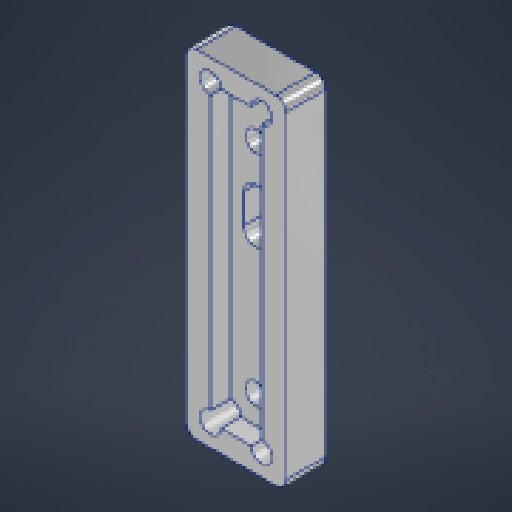
# Autodesk Inventor part: Zig
Saved by Autodesk Inventor 2024.3 (Build 283343000, 343)
## iProperties
Created: 2025-01-11
Part Number: Zig
Material: 알루미늄 6061
Document SubType Name: Modeling
Designer: ASUS
Density: 2.7 g/cm^3
Appearance: 알루미늄 - 평지
Author: ASUS
Autodesk Inventor part; units mm, degrees
ref_plane "YZ Plane" through (0, 0, 0) normal (1, 0, 0) x (0, 1, 0)
ref_plane "XZ Plane" through (0, 0, 0) normal (0, 1, 0) x (-1, 0, 0)
ref_plane "XY Plane" through (0, 0, 0) normal (0, 0, 1) x (1, 0, 0)
sketch "스케치1" plane through (0, 0, 0) normal (0, 0, 1) x (1, 0, 0)
  line L0 (-51.3249, -3.3936) -> (-51.3249, -32.7936) projected
  line L1 (-51.3249, -32.7936) -> (-56.3249, -32.7936) projected
  line L2 (-56.3249, -32.7936) -> (-56.3249, -3.3936) projected
  line L3 (-56.3249, -3.3936) -> (-51.3249, -3.3936) projected
  ellipse E0 centre (-53.8249, -30.0936) end of major axis (-54.8249, -30.0936) minor radius 1 projected
  ellipse E1 centre (-53.8249, -8.0936) end of major axis (-54.8249, -8.0936) minor radius 1 projected
  line L4 (5, 29.3999) -> (5, 0)
  line L5 (5, 0) -> (0, 0)
  line L6 (0, 0) -> (0, 29.3999)
  line L7 (0, 29.3999) -> (5, 29.3999)
  ellipse E2 centre (2.5, 2.7) end of major axis (1.5, 2.7) minor radius 1
  ellipse E3 centre (2.5, 24.7) end of major axis (1.5, 24.7) minor radius 1
  line L8 (5.06, -0.06) -> (5.06, 29.4599)
  line L9 (5.06, 29.4599) -> (-0.06, 29.4599)
  line L10 (-0.06, 29.4599) -> (-0.06, -0.06)
  line L11 (-0.06, -0.06) -> (5.06, -0.06)
  line L12 (2.5, 29.4599) -> (2.5, -0.06)
  line L13 (-2.5, -2.3) -> (7.5, -2.3)
  line L14 (7.5, -2.3) -> (7.5, 31.7)
  line L15 (7.5, 31.7) -> (-2.5, 31.7)
  line L16 (-2.5, 31.7) -> (-2.5, -2.3)
  line L17 (-2.5, -2.3) -> (7.5, 31.7) construction
  line L18 (7.5, -2.3) -> (-2.5, 31.7) construction
  circle A0 centre (2.5, 24.7) radius 1.05
  circle A1 centre (2.5, 2.7) radius 1.05
  point P0 (2.5, 14.7)
  dimension "d0" = 0.06
  dimension "d1" = 10
  dimension "d2" = 34
  dimension "d5" = 2.1
  dimension "d6" = 2.1
  constraints: 30 end point, 5 midpoint, 2 centre point, 2 coincident, 2 parallel, 1 horizontal, 1 perpendicular, 9 other
  measures "d0" distance between parallel lines of L4 L8
  measures "d1" distance of L15.end L14.end
  measures "d2" distance of L14.end L13.end
  measures "d5" diameter of A0
  measures "d6" diameter of A1
extrude "돌출1" add sketch "스케치1" along normal blind 2 contours L7 L12 L9 L8 L11 L5 L4 | L4 L5 L12 A1 A0 L7 | L12 A0 A1 L5 L6 L7 | L7 L6 L5 L12 L11 L10 L9 | A0 L12 E3 | L12 E3 A0 | A1 L12 E2 | L12 E2 A1 | L16 L15 L14 L13
sketch "스케치2" plane through (0, 0, 2) normal (0, 0, 1) x (1, 0, 0)
  line L0 (7.5, -2.3) -> (7.5, 31.7) projected
  line L1 (7.5, 31.7) -> (-2.5, 31.7) projected
  line L2 (-2.5, 31.7) -> (-2.5, -2.3) projected
  line L3 (-2.5, -2.3) -> (7.5, -2.3) projected
  ellipse E0 centre (2.5, 24.7) end of major axis (3.5, 24.7) minor radius 1 projected
  ellipse E1 centre (2.5, 2.7) end of major axis (3.5, 2.7) minor radius 1 projected
  line L4 (5, 29.3999) -> (5, 0)
  line L5 (0, 0) -> (0, 29.3999)
  line L6 (5.06, -0.06) -> (5.06, 29.4599)
  line L7 (2.5, 29.4599) -> (2.5, -0.06)
  line L8 (-2.5, 31.7) -> (-2.5, -2.3)
  line L9 (7.5, -2.3) -> (7.5, 31.7)
  line L10 (-2.5, -2.3) -> (7.5, 31.7) construction
  line L11 (7.5, -2.3) -> (-2.5, 31.7) construction
  line L12 (-0.06, 29.4599) -> (-0.06, -0.06)
  ellipse E2 centre (2.5, 24.7) end of major axis (1.5, 24.7) minor radius 1
  circle A0 centre (2.5, 24.7) radius 1.05
  line L13 (0, 29.3999) -> (5, 29.3999)
  line L14 (5.06, 29.4599) -> (-0.06, 29.4599)
  line L15 (7.5, 31.7) -> (-2.5, 31.7)
  ellipse E3 centre (2.5, 2.7) end of major axis (1.5, 2.7) minor radius 1
  circle A1 centre (2.5, 2.7) radius 1.05
  line L16 (5, 0) -> (0, 0)
  line L17 (-0.06, -0.06) -> (5.06, -0.06)
  line L18 (-2.5, -2.3) -> (7.5, -2.3)
  circle A2 centre (5.06, -0.06) radius 1.05
  circle A3 centre (-0.06, -0.06) radius 1.05
  circle A4 centre (-0.06, 29.4599) radius 1.05
  circle A5 centre (5.06, 29.4599) radius 1.05
  point P0 (2.5, 14.7)
  point P1 (4.01, 29.4599)
  point P2 (5.06, 28.4099)
  point P3 (5.06, 0.99)
  point P4 (4.01, -0.06)
  point P5 (0.99, -0.06)
  point P6 (-0.06, 0.99)
  point P7 (-0.06, 28.4099)
  point P8 (0.99, 29.4599)
  dimension "d17" = 0.06
  dimension "d18" = 10
  dimension "d19" = 34
  dimension "d20" = 2.1
  dimension "d21" = 2.1
  dimension "d22" = 2.1
  dimension "d23" = 2.1
  dimension "d24" = 2.1
  dimension "d25" = 2.1
  constraints: 30 end point, 6 centre point, 6 coincident, 5 midpoint, 2 parallel, 1 horizontal, 1 perpendicular, 7 other
  measures "d17" distance between parallel lines of L4 L6
  measures "d18" distance of L8.start L10.end
  measures "d19" distance of L10.end L11.start
  measures "d20" diameter of A0
  measures "d21" diameter of A1
  measures "d22" diameter of A2
  measures "d23" diameter of A3
  measures "d24" diameter of A4
  measures "d25" diameter of A5
extrude "돌출2" add sketch "스케치2" along normal blind 2
fillet "모깎기1" radius 1 4 edges at (7.5, 31.7, 2) (-2.5, 31.7, 2) (7.5, -2.3, 2) (-2.5, -2.3, 2)
sketch "스케치3" plane through (0, 0, 4) normal (0, 0, 1) x (1, 0, 0)
  line L0 (4.01, 29.4599) -> (0.99, 29.4599) projected
  arc A0 (0.99, 29.4599) -> (-0.06, 28.4099) centre (-0.06, 29.4599) ccw projected
  line L1 (-0.06, 28.4099) -> (-0.06, 0.99) projected
  arc A1 (-0.06, 0.99) -> (0.99, -0.06) centre (-0.06, -0.06) ccw projected
  line L2 (0.99, -0.06) -> (4.01, -0.06) projected
  arc A2 (4.01, -0.06) -> (5.06, 0.99) centre (5.06, -0.06) ccw projected
  line L3 (5.06, 0.99) -> (5.06, 28.4099) projected
  arc A3 (5.06, 28.4099) -> (4.01, 29.4599) centre (5.06, 29.4599) ccw projected
  ellipse E0 centre (2.5, 24.7) end of major axis (3.5, 24.7) minor radius 1 projected
  ellipse E1 centre (2.5, 2.7) end of major axis (3.5, 2.7) minor radius 1 projected
  point P0 (0, 0)
hole "구멍1" at (-0.06, -0.06, 4) at (5.06, -0.06, 4) at (-0.06, 29.4599, 4) at (5.06, 29.4599, 4) at (2.5, 2.7, 4) at (2.5, 24.7, 4) direction (0, 0, -1) diameter 2.1 end through all
sketch "스케치4" plane through (0, 0, 0) normal (0, 0, -1) x (-1, 0, 0)
  circle A0 centre (-2.5, 24.7) radius 1.05 projected
  circle A1 centre (-2.5, 2.7) radius 1.05 projected
  circle A2 centre (-5.06, 29.4599) radius 1.05 projected
  circle A3 centre (0.06, 29.4599) radius 1.05 projected
  circle A4 centre (-5.06, -0.06) radius 1.05 projected
  circle A5 centre (0.06, -0.06) radius 1.05 projected
  arc A6 (1.5, -2.3) -> (2.5, -1.3) centre (1.5, -1.3) ccw projected
  line L0 (2.5, 30.7) -> (2.5, -1.3) projected
  arc A7 (2.5, 30.7) -> (1.5, 31.7) centre (1.5, 30.7) ccw projected
  line L1 (-6.5, 31.7) -> (1.5, 31.7) projected
  arc A8 (-6.5, 31.7) -> (-7.5, 30.7) centre (-6.5, 30.7) ccw projected
  line L2 (-7.5, -1.3) -> (-7.5, 30.7) projected
  arc A9 (-7.5, -1.3) -> (-6.5, -2.3) centre (-6.5, -1.3) ccw projected
  line L3 (1.5, -2.3) -> (-6.5, -2.3) projected
  line L4 (-2.5, 24.7) -> (-2.5, 19.7)
  circle A10 centre (-2.5, 19.7) radius 1.25
  line L5 (-2.5, 19.7) -> (-2.5, 16.7) construction
  line L6 (-1.25, 19.7) -> (-1.25, 16.7)
  line L7 (-3.75, 16.7) -> (-3.75, 19.7)
  arc A11 (-1.25, 19.7) -> (-3.75, 19.7) centre (-2.5, 19.7) ccw
  arc A12 (-3.75, 16.7) -> (-1.25, 16.7) centre (-2.5, 16.7) ccw
  point P0 (0, 0)
  point P1 (-2.5, 18.2)
  dimension "d36" = 5
  dimension "d37" = 2.5
  dimension "d38" = 3
  constraints: 10 end point, 4 point on circle, 4 tangent, 3 centre point, 2 vertical, 1 coincident, 1 concentric, 1 midpoint, 1 parallel
  measures "d36" distance of L4.start L4.end
  measures "d37" diameter of A10
  measures "d38" distance of L5.start L5.end
extrude "돌출3" cut sketch "스케치4" against normal through all contours A10 | A10 L6 A12 L7
